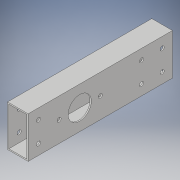
# Autodesk Inventor part: 1x2 7 in Beam Motor Mount
Saved by Autodesk Inventor 2018 (Build 220112000, 112)
## iProperties
Created: 2020-02-08
Part Number: 1x2 7 in Beam Motor Mount
Material: Generic
Document SubType Name: Modeling
Designer: Weeb No1
Density: 1 g/cm^3
Appearance: Default
Author: Weeb No1
Autodesk Inventor part; units mm, degrees
ref_plane "YZ Plane" through (0, 0, 0) normal (1, 0, 0) x (0, 1, 0)
ref_plane "XZ Plane" through (0, 0, 0) normal (0, 1, 0) x (-1, 0, 0)
ref_plane "XY Plane" through (0, 0, 0) normal (0, 0, 1) x (1, 0, 0)
sketch "Sketch1" plane through (0, 0, 0) normal (0, 0, 1) x (1, 0, 0)
  line L0 (0, 0) -> (25.4, 0)
  line L1 (25.4, 0) -> (25.4, 50.8)
  line L2 (25.4, 50.8) -> (0, 50.8)
  line L3 (0, 50.8) -> (0, 0)
  dimension "d0" = 25.4
  dimension "d1" = 50.8
  constraints: 8 end point, 2 parallel, 1 horizontal, 1 perpendicular
  measures "d0" distance of L2.end L1.end
  measures "d1" distance of L1.end L0.end
extrude "Extrusion1" add sketch "Sketch1" along normal blind 177.8
shell "Shell1" thickness 1.5875 removed faces 2 at (8.4667, 16.9333, 0) at (8.4667, 16.9333, 177.8)
hole "Hole1" at (25.4, 25.4, 114.3) direction (-1, 0, 0) diameter 28.575 end through all
sketch "Sketch2" plane through (25.4, 0, 0) normal (1, 0, 0) x (0, 0, -1)
  line L0 (-177.8, 1.5875) -> (-177.8, 49.2125) projected
  line L1 (-177.8, 25.4) -> (-114.3, 25.4)
  line L2 (-177.8, 25.4) -> (-114.3, 25.4) construction
  line L3 (-114.3, 25.4) -> (-88.9, 25.4)
  line L4 (-114.3, 25.4) -> (-139.7, 25.4)
  circle A0 centre (-139.7, 25.4) radius 2.5797
  circle A1 centre (-88.9, 25.4) radius 2.5797
  point P0 (0, 0)
  dimension "d14" = 63.5
  dimension "d16" = 25.4
  dimension "d17" = 25.4
  dimension "d18" = 5.1594
  dimension "d19" = 5.1594
  constraints: 8 end point, 3 horizontal, 2 centre point, 2 coincident, 1 collinear, 1 midpoint, 1 point on line
  measures "d14" distance of L1.start L1.end
  measures "d16" distance of L2.end L3.end
  measures "d17" distance of L2.end L4.end
  measures "d18" diameter of A0
  measures "d19" diameter of A1
extrude "Extrusion2" cut sketch "Sketch2" against normal blind 177.8
hole "Hole2" at (25.4, 38.1, 165.1) direction (-1, 0, 0) diameter 5.1594 end through all
hole "Hole3" at (25.4, 12.7, 165.1) direction (-1, 0, 0) diameter 5.1594 end through all
hole "Hole4" at (25.4, 38.1, 12.7) direction (-1, 0, 0) diameter 5.1594 end through all
hole "Hole5" at (25.4, 38.1, 38.1) direction (-1, 0, 0) diameter 5.1594 end through all
hole "Hole6" at (25.4, 12.7, 38.1) direction (-1, 0, 0) diameter 5.1594 end through all
hole "Hole7" at (25.4, 12.7, 12.7) direction (-1, 0, 0) diameter 5.1594 end through all
body "Solid1"
